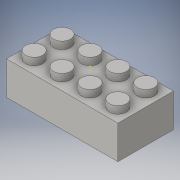
# Autodesk Inventor part: Lego Brick
Saved by Autodesk Inventor 2016 (Build 200138000, 138)
## iProperties
Created: 2016-02-04
Part Number: Lego Brick
Material: Generic
Document SubType Name: Modeling
Designer: yoruichin
Density: 1 g/cm^3
Appearance: Default
Author: yoruichin
Autodesk Inventor part; units mm, degrees
ref_plane "YZ Plane" through (0, 0, 0) normal (1, 0, 0) x (0, 1, 0)
ref_plane "XZ Plane" through (0, 0, 0) normal (0, 1, 0) x (-1, 0, 0)
ref_plane "XY Plane" through (0, 0, 0) normal (0, 0, 1) x (1, 0, 0)
sketch "Sketch1" plane through (0, 0, 0) normal (0, 0, 1) x (1, 0, 0)
  line L0 (-15.978, -4.8) -> (15.978, -4.8)
  line L1 (15.978, -4.8) -> (15.978, 4.8)
  line L2 (15.978, 4.8) -> (-15.978, 4.8)
  line L3 (-15.978, 4.8) -> (-15.978, -4.8)
  line L4 (-15.978, -4.8) -> (15.978, 4.8) construction
  line L5 (15.978, -4.8) -> (-15.978, 4.8) construction
  point P0 (0, 0)
  dimension "d0" = 31.956
  dimension "d1" = 9.6
  constraints: 12 end point, 2 midpoint, 2 parallel, 1 horizontal, 1 perpendicular
  measures "d0" distance of L2.end L1.end
  measures "d1" distance of L1.end L0.end
extrude "Extrusion1" add sketch "Sketch1" along normal mid plane 15.928
sketch "Sketch2" plane through (-15.978, 4.8, 7.964) normal (0, 1, 0) x (1, 0, 0)
  circle A0 centre (3.957, 3.957) radius 2.45
  point P0 (15.978, 7.964)
  dimension "d4" = 4.9
  constraints: 1 centre point
  measures "d4" diameter of A0
extrude "Extrusion2" add sketch "Sketch2" along normal blind 2.1
pattern_linear "Rectangular Pattern1" count 4 spacing 8.014 along (1, 0, 0) of "Extrusion2"
mirror "Mirror1" about plane through (0, 0, 0) normal (0, 0, 1) of "Extrusion2", "Rectangular Pattern1"
sketch "Sketch3" plane through (-12.021, 6.9, 4.007) normal (0, 1, 0) x (1, 0, 0)
  point P0 (12.021, 4.007)
shell "Shell1" thickness 1.557 removed faces 1 at (-5.326, -4.8, 2.6547)
sketch "Sketch4" plane through (-15.978, -4.8, 7.964) normal (0, -1, 0) x (1, 0, 0)
  point P0 (15.978, -7.964)
sketch "Sketch6" plane through (-14.421, 3.243, -6.407) normal (0, -1, 0) x (1, 0, 0)
  circle A0 centre (22.435, 6.407) radius 3.267
  circle A1 centre (22.435, 6.407) radius 2.467
  point P0 (14.421, 6.407)
  point P1 (30.399, -1.557)
  dimension "d13" = 6.534
  dimension "d14" = 0.8
  constraints: 2 centre point
  measures "d13" diameter of A0
  measures "d14" radial gap between concentric circles of A0 A1
extrude "Extrusion3" add sketch "Sketch6" along normal blind 3
pattern_linear "Rectangular Pattern2" count 3 spacing 8.014 along (-1, 0, 0) of "Extrusion3"
body "Solid1"
